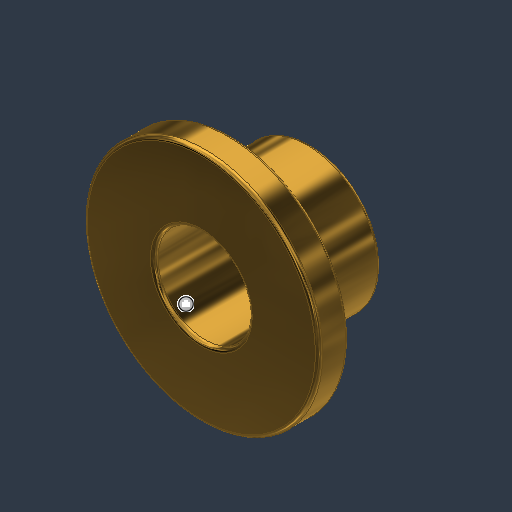
# Autodesk Inventor part: BUSHING,SHAFT,END_EFFECTOR,ARM
Saved by Autodesk Inventor 2024.3 (Build 283343000, 343)
## iProperties
Category: _
Manager: _
ILogicPurgeVersion: 0.0.0.0
OnSaveVersion: 2.2.20.20
Created: 2025-03-14
Part Number: BUSHING,SHAFT,END_EFFECTOR,ARM
Checked By: 00
Engr Approved By: _
User Status: Work In Process
Material: Brass, Soft Yellow
Description: STANDARD (mm)
Document SubType Name: Modeling
Mfg Approved By: Stephen.Oerton
Designer: John Thibert
Manufacturer: Standard
Standards Organization: Custom
Density: 8.47 g/cm^3
Appearance: Brass - Satin
Mass: 4.63375 g
Surface Area: 7.18678 cm^2
Volume: 0.547078 cm^3
CN_MASS: 0.0
CN_SERVICEABLE: _
FIRST_DESCRIPTION: _
SECOND_DESCRIPTION: _
THIRD_DESCRIPTION: _
ModelCat: Uncategorized
Subject: _
Author: John Thibert
Keywords: -
Revision Number: A
Autodesk Inventor part; units mm, degrees
ref_plane "YZ Plane" through (0, 0, 0) normal (1, 0, 0) x (0, 1, 0)
ref_plane "XZ Plane" through (0, 0, 0) normal (0, 1, 0) x (-1, 0, 0)
ref_plane "XY Plane" through (0, 0, 0) normal (0, 0, 1) x (1, 0, 0)
sketch "Sketch2" plane through (0, 0, 0) normal (0, 1, 0) x (-1, 0, 0)
  line L0 (0, -8.8392) -> (0, 1.4732) construction
  line L1 (-7.9375, 0) -> (-3.175, 0)
  line L2 (-3.175, 0) -> (-3.175, -7.366)
  line L3 (-3.175, -7.366) -> (-4.7625, -7.366)
  line L4 (-4.7625, -7.366) -> (-4.7625, -2.032)
  line L5 (-4.7625, -2.032) -> (-7.9375, -2.032)
  line L6 (-7.9375, -2.032) -> (-7.9375, 0)
  point P0 (0, 0)
  dimension "d0" = 2.032
  dimension "d1" = 6.35
  dimension "d2" = 9.525
  dimension "d5" = 15.875
  dimension "d9" = 7.366
  constraints: 12 end point, 5 perpendicular, 1 horizontal, 1 point on line
  measures "d0" distance between parallel lines of L5 L1
  measures "d1" diameter of L2 L0
  measures "d2" diameter of L4 L0
  measures "d5" diameter of L6 L0
  measures "d9" distance between parallel lines of L3 L1
revolve "Revolution1" add sketch "Sketch2" angle 360 about axis through (0, 0, 0) along (0, 0, 1)
fillet "Fillet1" radius 0.254 6 edges at (-4.7625, 0, -2.032) (-7.9375, 0, -2.032) (-7.9375, 0, 0) (-4.7625, 0, -7.366) (-3.175, 0, -7.366) (-3.175, 0, 0)
body "Solid1"
